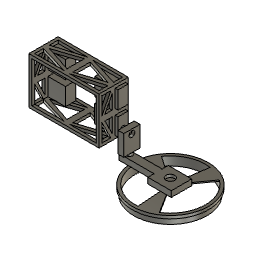
initial ideas and model (Autodesk Fusion 360 design; units mm, degrees)
Autodesk Fusion 360 part; units mm, degrees
note: some values were not read from the file. Set by a fixed rule: which sketch regions a step uses.
sketch "Sketch1" plane through (0, 0, 0) normal (0, 1, 0) x (1, 0, 0)
  line L0 (-60, -40) -> (60, -40)
  line L1 (60, -40) -> (60, 40)
  line L2 (60, 40) -> (-60, 40)
  line L3 (-60, 40) -> (-60, -40)
  dimension "d1" = 120
  dimension "d2" = 80
  dimension "d3" = 40
  dimension "d4" = 60
  constraint horizontal L0
  constraint vertical L1
  constraint horizontal L2
  constraint vertical L3
  measures "d1" distance of L0.start L0.end
  measures "d2" distance of L0.start L2.end
  measures "d3" distance of origin L0
  measures "d4" distance of origin L3
extrude "Extrude1" add sketch "Sketch1" along normal blind 50 makes body 1
sketch "Sketch2" plane through (0, 50, 0) normal (0, 1, 0) x (-1, 0, 0)
  line L0 (60, -40) -> (60, 40)
  line L1 (60, 40) -> (-60, 40)
  line L2 (-60, 40) -> (-60, -40)
  line L3 (-60, -40) -> (60, -40)
  line L4 (-55, 35) -> (55, 35)
  line L5 (55, 35) -> (55, -35)
  line L6 (55, -35) -> (-55, -35)
  line L7 (-55, -35) -> (-55, 35)
  constraint horizontal L4
  constraint vertical L5
  constraint horizontal L6
  constraint vertical L7
extrude "Extrude2" cut sketch "Sketch2" against normal blind 50 contours L4 L5 L6 L7 bodies 1
sketch "Sketch3" plane through (60, 0, 0) normal (1, 0, 0) x (0, 1, 0)
  line L0 (0, 40) -> (0, -40)
  line L1 (0, -40) -> (50, -40)
  line L2 (50, -40) -> (50, 40)
  line L3 (50, 40) -> (0, 40)
  line L4 (45, -35) -> (30, -35)
  line L5 (30, -35) -> (45, -5)
  line L6 (45, -5) -> (45, -35)
  line L7 (20, -35) -> (5, -35)
  line L8 (5, -35) -> (5, -5)
  line L9 (5, -5) -> (20, -35)
  line L10 (10, -5) -> (22.5311, -30.0622)
  line L11 (22.5245, -5) -> (10, -5)
  line L12 (40, -5) -> (27.4689, -5)
  line L13 (27.4689, -30.0622) -> (40, -5)
  line L14 (45, 5) -> (45, 35)
  line L15 (45, 35) -> (30, 35)
  line L16 (45, 5) -> (45, 35)
  line L17 (45, 35) -> (30, 35)
  line L18 (30, 35) -> (45, 5)
  line L19 (40, 5) -> (27.4689, 5)
  line L20 (22.5245, 5) -> (10, 5)
  line L21 (10, 5) -> (22.5245, 30.049)
  line L22 (5, 5) -> (20, 35)
  line L23 (20, 35) -> (5, 35)
  line L24 (5, 35) -> (5, 5)
  line L25 (22.5311, -30.0622) -> (22.5245, -30.0622)
  line L26 (27.4689, 30.049) -> (27.4689, 5)
  line L27 (27.4689, -5) -> (27.4689, -30.0622)
  line L28 (22.5245, -30.0622) -> (22.5245, -5)
  line L29 (22.5245, 5) -> (22.5245, 30.049)
  line L30 (40, 5) -> (27.4689, 30.049)
  constraint horizontal L4
  constraint perpendicular L4 L6
  constraint perpendicular L6 L7
  constraint perpendicular L7 L8
  constraint parallel L9 L10
  constraint horizontal L25
  constraint vertical L28
  constraint vertical L26
  constraint coincident L12.end L26
  constraint collinear L26 L27
  constraint collinear L28 L29
extrude "Extrude3" cut sketch "Sketch3" against normal blind 120 contours L4 L5 L6 | L7 L8 L9 | L10 L11 L28 | L12 L13 L27 | L14 L15 L16 L17 L18 | L19 L26 L30 | L20 L21 L29 | L22 L23 L24 bodies 1
sketch "Sketch4" plane through (0, 0, -40) normal (0, 0, -1) x (1, 0, 0)
  line L0 (60, 0) -> (-60, 0)
  line L1 (-60, 0) -> (-60, -50)
  line L2 (-60, -50) -> (60, -50)
  line L3 (60, -50) -> (60, 0)
  line L4 (0, 25) -> (0, -70)
  line L5 (-75, -25) -> (70, -25)
  line L6 (-55, -5) -> (-55, -20)
  line L7 (-55, -20) -> (-5, -5)
  line L8 (-5, -5) -> (-55, -5)
  line L9 (-50, -25) -> (-5, -10)
  line L10 (-5, -10) -> (-5, -25)
  line L11 (5, -5) -> (55, -5)
  line L12 (55, -5) -> (55, -20)
  line L13 (55, -20) -> (5, -5)
  line L14 (50, -25) -> (5, -10)
  line L15 (5, -10) -> (5, -25)
  line L16 (-55, -45) -> (-55, -30)
  line L17 (5, -45) -> (55, -45)
  line L18 (55, -30) -> (5, -45)
  line L19 (-55, -30) -> (-5, -45)
  line L20 (-5, -45) -> (-55, -45)
  line L21 (55, -45) -> (55, -30)
  line L22 (-50, -25) -> (-5, -40)
  line L23 (-5, -40) -> (-5, -25)
  line L24 (5, -40) -> (5, -25)
  line L25 (50, -25) -> (5, -40)
  point P0 (60, -50)
  point P1 (0, -50)
  constraint vertical L4
  constraint horizontal L5
  constraint vertical L6
  constraint perpendicular L6 L8
  constraint coincident L5 L9.start
  constraint coincident L5 L10.end
  constraint perpendicular L5 L10
  constraint symmetric L4 L6.start L11.end
  constraint symmetric L4 L6.end L12.end
  constraint symmetric L4 L7.end L11.start
  constraint symmetric L4 L9.start L14.start
  constraint symmetric L4 L9.end L14.end
  constraint symmetric L4 L10.end L15.end
  constraint symmetric origin L5 P1
  constraint symmetric L0.start L5 P0
  constraint symmetric L5 L6.start L16.start
  constraint symmetric L5 L6.end L16.end
  constraint symmetric L5 L7.end L19.end
  constraint symmetric L5 L9.start L22.start
  constraint symmetric L5 L9.end L22.end
  constraint symmetric L5 L10.end L23.end
  constraint symmetric L5 L11.start L17.start
  constraint symmetric L5 L11.end L17.end
  constraint symmetric L5 L12.end L18.start
  constraint symmetric L5 L14.start L25.start
  constraint symmetric L5 L14.end L24.start
  constraint symmetric L5 L15.end L24.end
extrude "Extrude4" cut sketch "Sketch4" against normal blind 80 contours L5 L24 L25 | L5 L14 L15 | L5 L22 L23 | L5 L9 L10 | L6 L7 L8 | L11 L12 L13 | L16 L19 L20 | L17 L18 L21 bodies 1
sketch "Sketch5" plane through (55, 0, 0) normal (-1, 0, 0) x (0, -1, 0)
  line L0 (-22.5245, 30.049) -> (-10, 5)
  line L1 (-10, 5) -> (-22.5245, 5)
  line L2 (-22.5245, 5) -> (-22.5245, 30.049)
  line L3 (-27.4689, 5) -> (-40, 5)
  line L4 (-40, 5) -> (-27.4689, 30.049)
  line L5 (-27.4689, 30.049) -> (-27.4689, 5)
  line L6 (-40, -5) -> (-27.4689, -5)
  line L7 (-27.4689, -5) -> (-27.4689, -30.0622)
  line L8 (-27.4689, -30.0622) -> (-40, -5)
  line L9 (-10, -5) -> (-22.5245, -30.049)
  line L10 (-22.5245, -30.049) -> (-22.5245, -5)
  line L11 (-22.5245, -5) -> (-10, -5)
  line L12 (-5, -5) -> (-5, -35)
  line L13 (-5, -35) -> (0, -35)
  line L14 (0, -35) -> (0, 35)
  line L15 (0, 35) -> (-5, 35)
  line L16 (-5, 35) -> (-5, 5)
  line L17 (-5, 5) -> (-20, 35)
  line L18 (-20, 35) -> (-30, 35)
  line L19 (-30, 35) -> (-45, 5)
  line L20 (-45, 5) -> (-45, 35)
  line L21 (-45, 35) -> (-50, 35)
  line L22 (-50, 35) -> (-50, -35)
  line L23 (-50, -35) -> (-45, -35)
  line L24 (-45, -35) -> (-45, -5)
  line L25 (-45, -5) -> (-30, -35)
  line L26 (-30, -35) -> (-20, -35)
  line L27 (-20, -35) -> (-5, -5)
  line L28 (-45, -5) -> (-27.3665, -5)
  line L29 (-27.3665, -5) -> (-27.3665, -35)
  line L30 (-27.3665, -35) -> (-45, -35)
  line L31 (-45, -35) -> (-45, -5)
  line L32 (-22.5245, -5) -> (-5, -5)
  line L33 (-5, -5) -> (-5, -35)
  line L34 (-5, -35) -> (-22.5245, -35)
  line L35 (-22.5245, -35) -> (-22.5245, -5)
  line L36 (-23.0946, 35) -> (-5, 35)
  line L37 (-5, 35) -> (-5, 5)
  line L38 (-5, 5) -> (-23.0946, 5)
  line L39 (-23.0946, 5) -> (-23.0946, 35)
  line L40 (-45, 35) -> (-27.4689, 35)
  line L41 (-27.4689, 35) -> (-27.4689, 5)
  line L42 (-27.4689, 5) -> (-45, 5)
  line L43 (-45, 5) -> (-45, 35)
  constraint horizontal L28
  constraint vertical L29
  constraint horizontal L30
  constraint vertical L31
  constraint coincident L26 L29.end
  constraint coincident L24.end L25.start
  constraint horizontal L32
  constraint vertical L33
  constraint horizontal L34
  constraint vertical L35
  constraint coincident L12.end L13.start
  constraint coincident L10.end L11.start
  constraint horizontal L36
  constraint vertical L37
  constraint horizontal L38
  constraint vertical L39
  constraint coincident L16.end L17.start
  constraint coincident L18 L36.start
  constraint horizontal L40
  constraint vertical L41
  constraint horizontal L42
  constraint vertical L43
  constraint coincident L3.start L5.end
  constraint coincident L20.end L21.start
extrude "Extrude5" add sketch "Sketch5" along normal blind 30 and the other way blind 10 contours L4 L18 L19 L40 L41 L42 | L19 L20 L40 L43 | L3 L4 L5 L41 L42 | L7 L8 L25 L26 L28 L29 L30 | L24 L25 L30 L31 | L6 L7 L8 L28 bodies 1
sketch "Sketch6" plane through (-55, 0, 0) normal (1, 0, 0) x (0, 1, 0)
  line L0 (10, -5) -> (22.5245, -5)
  line L1 (22.5245, -5) -> (22.5245, -30.049)
  line L2 (22.5245, -30.049) -> (10, -5)
  line L3 (20, -35) -> (30, -35)
  line L4 (30, -35) -> (45, -5)
  line L5 (45, -5) -> (45, -35)
  line L6 (45, -35) -> (50, -35)
  line L7 (50, -35) -> (50, 35)
  line L8 (50, 35) -> (45, 35)
  line L9 (45, 35) -> (45, 5)
  line L10 (45, 5) -> (30, 35)
  line L11 (30, 35) -> (20, 35)
  line L12 (20, 35) -> (5, 5)
  line L13 (5, 5) -> (5, 35)
  line L14 (5, 35) -> (0, 35)
  line L15 (0, 35) -> (0, -35)
  line L16 (0, -35) -> (5, -35)
  line L17 (5, -35) -> (5, -5)
  line L18 (5, -5) -> (20, -35)
  line L19 (27.4689, 30.049) -> (40, 5)
  line L20 (40, 5) -> (27.4689, 5)
  line L21 (27.4689, 5) -> (27.4689, 30.049)
  line L22 (40, -5) -> (27.4689, -30.0622)
  line L23 (27.4689, -30.0622) -> (27.4689, -5)
  line L24 (27.4689, -5) -> (40, -5)
  line L25 (22.5245, 5) -> (10, 5)
  line L26 (10, 5) -> (22.5245, 30.049)
  line L27 (22.5245, 30.049) -> (22.5245, 5)
  line L28 (27.4689, 35) -> (45, 35)
  line L29 (45, 35) -> (45, 5)
  line L30 (45, 5) -> (27.4689, 5)
  line L31 (27.4689, 5) -> (27.4689, 35)
  line L32 (27.4689, -5) -> (45, -5)
  line L33 (45, -5) -> (45, -35)
  line L34 (45, -35) -> (27.4689, -35)
  line L35 (27.4689, -35) -> (27.4689, -5)
  constraint horizontal L28
  constraint vertical L29
  constraint horizontal L30
  constraint vertical L31
  constraint coincident L9.end L10.start
  constraint coincident L11 L28.start
  constraint horizontal L32
  constraint vertical L33
  constraint horizontal L34
  constraint vertical L35
  constraint coincident L5.end L6.start
  constraint coincident L23.end L24.start
extrude "Extrude6" add sketch "Sketch6" along normal blind 30 and the other way blind 10 contours L3 L4 L22 L32 L34 L35 | L4 L5 L33 L34 | L22 L23 L24 L32 L35 | L9 L10 L28 L29 | L10 L11 L19 L28 L30 L31 | L19 L20 L21 L30 L31 bodies 1
sketch "Sketch7" plane through (65, 0, 0) normal (1, 0, 0) x (0, 1, 0)
  line L0 (27.3665, -35) -> (45, -35)
  line L1 (45, -35) -> (45, -5)
  line L2 (45, -5) -> (27.3665, -5)
  line L3 (27.3665, -5) -> (27.3665, -35)
  circle A0 centre (36.1832, -27.2154) radius 5
  dimension "d21" = 10
  measures "d21" diameter of A0
extrude "Extrude7" add sketch "Sketch7" along normal blind 10 separate body contours A0 makes body 2
sketch "Sketch8" plane through (75, 0, 0) normal (1, 0, 0) x (0, 1, 0)
  circle A0 centre (36.1832, -27.2154) radius 5
  line L0 (27.3489, -19.8088) -> (45, -19.8088)
  line L1 (45, -19.8088) -> (45, -55)
  line L2 (45, -55) -> (27.3489, -55)
  line L3 (27.3489, -55) -> (27.3489, -19.8088)
  constraint horizontal L0
  constraint vertical L1
  constraint horizontal L2
  constraint vertical L3
extrude "Extrude8" add sketch "Sketch8" along normal blind 5 and the other way blind 5 bodies 2
extrude "Extrude9" add 1 faces at (73.3333, 45, -31.5392) along direction (0, 1, 0) blind 5 on bodies 2 bodies 2
extrude "Extrude10" add 1 faces at (76.6667, 27.3489, -31.5392) along direction (0, -1, 0) blind 5 on bodies 2 bodies 2
sketch "Sketch9" plane through (0, 0, -55) normal (0, 0, -1) x (1, 0, 0)
  line L0 (80, -50) -> (80, -22.3489)
  line L1 (80, -22.3489) -> (70, -22.3489)
  line L2 (70, -22.3489) -> (70, -50)
  line L3 (70, -50) -> (80, -50)
  circle A0 centre (75, -37) radius 5
  constraint tangent L2 A0
extrude "Extrude11" add sketch "Sketch9" along normal blind 10 contours A0 bodies 2
sketch "Sketch10" plane through (0, 0, -65) normal (0, 0, -1) x (1, 0, 0)
  circle A0 centre (75, -37) radius 5
  line L0 (125, -53.5) -> (125, -18.5)
  line L1 (125, -43) -> (65, -43)
  line L2 (65, -43) -> (65, -29)
  line L3 (65, -29) -> (125, -29)
  line L4 (125, -29) -> (125, -43)
  circle A1 centre (145, -37) radius 7.5
  line L5 (125, -53.5) -> (165, -53.5)
  line L6 (125, -18.5) -> (165, -18.5)
  line L7 (165, -53.5) -> (165, -18.5)
  dimension "d34" = 15
  dimension "d35" = 60
  dimension "d36" = 10
  dimension "d37" = 40
  dimension "d38" = 40
  dimension "d39" = 35
  dimension "d40" = 10.5
  dimension "d41" = 29
  dimension "d42" = 43
  dimension "d43" = 20
  constraint vertical L0
  constraint horizontal L1
  constraint vertical L2
  constraint horizontal L3
  constraint vertical L4
  constraint coincident L0 L1.start
  constraint perpendicular L0 L5
  constraint perpendicular L0 L6
  measures "d34" diameter of A1
  measures "d35" distance of L1.start L1.end
  measures "d36" distance of A0.centre L2
  measures "d37" distance of L0.start L5.end
  measures "d38" distance of L0.end L6.end
  measures "d39" distance of L5.end L6.end
  measures "d40" distance of L3 L6
  measures "d41" distance of origin L3
  measures "d42" distance of origin L1
  measures "d43" distance of A1.centre L7
extrude "Extrude12" add sketch "Sketch10" along normal blind 10 separate body contours A1 makes body 3
extrude "Extrude13" add sketch "Sketch10" along normal blind 5 and the other way blind 5 bodies 2 3
sketch "Sketch11" plane through (0, 0, -70) normal (0, 0, -1) x (1, 0, 0)
  circle A0 centre (75, -37) radius 5
  circle A1 centre (145, -37) radius 7.5
  line L0 (125, -53.5) -> (165, -53.5)
  line L1 (165, -53.5) -> (165, -18.5)
  line L2 (165, -18.5) -> (125, -18.5)
  line L3 (125, -18.5) -> (125, -29)
  line L4 (125, -29) -> (65, -29)
  line L5 (65, -29) -> (65, -43)
  line L6 (65, -43) -> (125, -43)
  line L7 (125, -43) -> (125, -53.5)
  circle A2 centre (145, -37) radius 65
  circle A3 centre (145, -37) radius 60
  line L8 (180.1394, -85.6335) -> (145, -37)
  line L9 (145, -37) -> (153.5051, -96.3941)
  line L10 (145, -37) -> (176.9644, 13.7767)
  line L11 (145, -37) -> (149.2525, 22.8491)
  line L12 (145, -37) -> (95.6347, -71.1037)
  line L13 (145, -37) -> (85, -37)
  dimension "d50" = 120
  constraint concentric A1 A2
  constraint tangent A0 A2
  constraint concentric A2 A3
  constraint coincident A3 L8.start
  constraint coincident A1.centre A2.centre
  constraint coincident A3 L9.end
  constraint coincident A3 L10.end
  constraint coincident A3 L11.end
  constraint coincident A3 L12.end
  constraint coincident A3 L13.end
  constraint horizontal L13
  measures "d50" diameter of A3
extrude "Extrude14" add sketch "Sketch11" along normal blind 2 contours A1 L6 L7 A3 L12 L13 | L6 L7 A3 L12 | L2 A3 L10 L11 | A1 L2 L10 L11 | L0 A3 L8 L9 | A1 L0 L8 L9 bodies 2
extrude "Extrude15" add sketch "Sketch11" along normal blind 15 contours L4 L6 A2 A3 | L4 L6 A2 A3 bodies 2
sketch "Sketch12" plane through (0, 0, -85) normal (0, 0, -1) x (1, 0, 0)
  circle A0 centre (145, -37) radius 60
  circle A1 centre (145, -37) radius 65
  circle A2 centre (145, -37) radius 62.5
  dimension "d55" = 125
  constraint concentric A0 A2
  measures "d55" diameter of A2
extrude "Extrude16" cut sketch "Sketch12" against normal blind 10 contours A1 bodies 2
